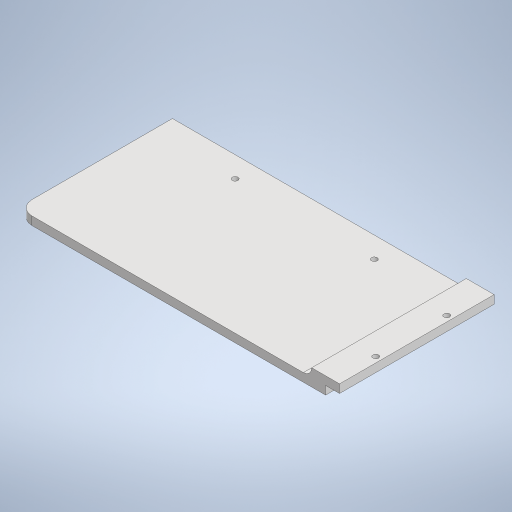
# Autodesk Inventor part: 底板_A
Saved by Autodesk Inventor 2023 (Build 270158000, 158)
## iProperties
Created: 2024-05-21
Part Number: 底板_A
Material: 常规
Document SubType Name: Modeling
Designer: Nitrene.P.L
Density: 1 g/cm^3
Appearance: 默认
Author: Nitrene.P.L
Autodesk Inventor part; units mm, degrees
ref_plane "YZ Plane" through (0, 0, 0) normal (1, 0, 0) x (0, 1, 0)
ref_plane "XZ Plane" through (0, 0, 0) normal (0, 1, 0) x (-1, 0, 0)
ref_plane "XY Plane" through (0, 0, 0) normal (0, 0, 1) x (1, 0, 0)
sketch "草图1" plane through (0, 0, 0) normal (0, 1, 0) x (-1, 0, 0)
  line L0 (110.5, 55.5) -> (-110.5, 55.5)
  line L1 (-110.5, 55.5) -> (-110.5, -55.5)
  line L2 (-110.5, -55.5) -> (110.5, -55.5)
  line L3 (110.5, -55.5) -> (110.5, 55.5)
  line L4 (0, 7.5575) -> (0, -11)
  line L5 (8.5019, 0) -> (-7, 0)
  point P0 (0, 0)
  dimension "d0" = 221
  dimension "d1" = 111
  constraints: 12 end point, 2 horizontal, 2 parallel, 2 vertical, 1 perpendicular, 2 other
  measures "d0" distance of L2.end L1.end
  measures "d1" distance of L1.end L0.end
extrude "拉伸1" add sketch "草图1" along normal blind 6
fillet "圆角1" radius 10.1 1 edges at (-110.5, 3, 55.5)
sketch "草图2" plane through (0, 6, 0) normal (0, 1, 0) x (1, 0, 0)
  line L0 (110.5, 55.5) -> (-110.5, 55.5) projected
  line L1 (100.5, 55.5) -> (120.5, 55.5)
  line L2 (120.5, 55.5) -> (120.5, -55.5)
  line L3 (120.5, -55.5) -> (100.5, -55.5)
  line L4 (100.5, -55.5) -> (100.5, 55.5)
  line L5 (110.5, -55.5) -> (110.5, 55.5) projected
  line L6 (-100.4, -55.5) -> (110.5, -55.5) projected
  circle A0 centre (116.5, 25.5) radius 2.1
  circle A1 centre (116.5, -25.5) radius 2.1
  point P0 (0, 0)
  dimension "d5" = 20
  dimension "d6" = 10
  dimension "d7" = 4.2
  dimension "d8" = 4.2
  dimension "d9" = 4
  dimension "d10" = 4
  dimension "d11" = 30
  dimension "d12" = 30
  constraints: 8 end point, 2 centre point, 2 parallel, 1 collinear, 1 horizontal, 1 perpendicular, 1 point on line
  measures "d5" distance of L2.end L3.end
  measures "d6" distance between parallel lines of L5 L4
  measures "d7" diameter of A0
  measures "d8" diameter of A1
  measures "d9" distance from line of L2 A0.centre
  measures "d10" distance from line of L2 A1.centre
  measures "d11" distance from line of L1 A0.centre
  measures "d12" distance from line of L3 A1.centre
extrude "拉伸2" add sketch "草图2" along normal blind 6
fillet "圆角2" radius 6 1 edges at (100.5, 6, 0)
sketch "草图3" plane through (0, 0, 0) normal (0, -1, 0) x (1, 0, 0)
  circle A0 centre (-50.5, -40.5) radius 2.1
  circle A1 centre (49.5, -40.5) radius 2.1
  line L0 (110.5, -55.5) -> (-110.5, -55.5) projected
  line L1 (-110.5, -55.5) -> (-110.5, 45.4) projected
  point P0 (0, 0)
  dimension "d16" = 4.2
  dimension "d17" = 4.2
  dimension "d18" = 15
  dimension "d19" = 15
  dimension "d20" = 60
  dimension "d21" = 100
  constraints: 2 centre point
  measures "d16" diameter of A0
  measures "d17" diameter of A1
  measures "d18" distance from line of L0 A0.centre
  measures "d19" distance from line of L0 A1.centre
  measures "d20" distance from line of L1 A0.centre
  measures "d21" distance of A0.centre A1.centre
extrude "拉伸3" cut sketch "草图3" against normal blind 10
